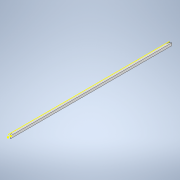
# Autodesk Inventor part: Main
Saved by Autodesk Inventor 2020.1 (Build 241239000, 239)
## iProperties
Created: 2020-02-04
Part Number: Main
Material: Generic
Document SubType Name: Modeling
Designer: super
Density: 1 g/cm^3
Appearance: Default
Author: super
Autodesk Inventor part; units mm, degrees
ref_plane "YZ Plane" through (0, 0, 0) normal (1, 0, 0) x (0, 1, 0)
ref_plane "XZ Plane" through (0, 0, 0) normal (0, 1, 0) x (-1, 0, 0)
ref_plane "XY Plane" through (0, 0, 0) normal (0, 0, 1) x (1, 0, 0)
sketch "Sketch1" plane through (0, 0, 0) normal (0, 1, 0) x (-1, 0, 0)
  line L0 (0, 0) -> (0, -412)
  line L1 (0, -412) -> (6.35, -412)
  line L2 (6.35, -412) -> (6.35, 0)
  line L3 (6.35, 0) -> (0, 0)
  dimension "d0" = 412
  dimension "d1" = 6.35
  constraints: 8 end point, 3 perpendicular, 1 vertical
  measures "d0" distance of L0.start L0.end
  measures "d1" distance of L0.end L1.end
extrude "Extrusion1" add sketch "Sketch1" along normal blind 6.35
sketch "Sketch2" plane through (0, 6.35, 0) normal (0, 1, 0) x (1, 0, 0)
  point P0 (0, 0)
sketch "Sketch3" plane through (-6.35, 0, -412) normal (-1, 0, 0) x (0, 0, 1)
  line L0 (412, 6.35) -> (0, 6.35) projected
  point P0 (412, 0)
sketch "Sketch4" plane through (-6.35, 0, -412) normal (-1, 0, 0) x (0, 0, 1)
  line L0 (412, 6.35) -> (403.5733, 0)
  line L1 (412, 0) -> (0, 0) projected
  line L2 (412, 6.35) -> (422.5514, 6.35) construction
  line L3 (403.5733, 0) -> (412, 0)
  line L4 (412, 0) -> (412, 6.35)
  dimension "d6" = 143
  constraints: 8 end point, 2 point on line, 1 collinear, 1 equal length, 1 horizontal, 1 perpendicular
  measures "d6" angle of L0 L2
extrude "Extrusion2" cut sketch "Sketch4" against normal blind 10
sketch "Sketch5" plane through (-6.35, 0, -412) normal (-1, 0, 0) x (0, 0, 1)
  line L0 (0, 6.35) -> (8.4267, 0)
  line L1 (0, 6.35) -> (10.5514, 6.35) construction
  line L2 (8.4267, 0) -> (0, 0)
  line L3 (0, 6.35) -> (412, 6.35) projected
  line L4 (0, 0) -> (0, 6.35)
  point P0 (412, 0)
  dimension "d9" = 37
  constraints: 8 end point, 1 equal length, 1 horizontal, 1 parallel, 1 perpendicular
  measures "d9" angle of L0 L1
extrude "Extrusion3" cut sketch "Sketch5" against normal blind 10
sketch "Sketch6" plane through (-6.35, 0, -403.5733) normal (-1, 0, 0) x (0, 0, 1)
  line L0 (403.5733, 6.35) -> (-8.4267, 6.35) projected
  line L1 (403.5733, 6.35) -> (403.5733, 0)
  line L2 (403.5733, 6.35) -> (395.1465, 0) projected
  line L3 (403.5733, 0) -> (395.1465, 0)
  line L4 (395.1465, 0) -> (403.5733, 6.35)
  constraints: 6 end point, 1 collinear, 1 perpendicular, 1 vertical
extrude "Extrusion4" add sketch "Sketch6" against normal blind 6.35
sketch "Sketch7" plane through (-6.35, 6.35, -412) normal (-1, 0, 0) x (0, 0, 1)
  line L0 (8.4267, -6.35) -> (412, -6.35) projected
  line L1 (8.4267, -6.35) -> (0, -6.35)
  line L2 (0, 0) -> (412, 0) projected
  line L3 (0, -6.35) -> (0, 0)
  line L4 (0, 0) -> (8.4267, -6.35)
  constraints: 6 end point, 1 horizontal, 1 perpendicular
extrude "Extrusion5" add sketch "Sketch7" against normal blind 6.35
sketch "Sketch8" plane through (0, 6.35, 0) normal (0, 1, 0) x (1, 0, 0)
  line L0 (-6.35, 0) -> (0, 0) projected
  line L1 (0, 0) -> (-6.35, 8.4267)
  line L2 (0, 0) -> (10.5514, 0) construction
  line L3 (-6.35, 8.4267) -> (-6.35, 0)
  line L4 (-6.35, 0) -> (0, 0)
  dimension "d16" = 127
  constraints: 8 end point, 1 collinear, 1 equal length, 1 horizontal, 1 perpendicular
  measures "d16" angle of L2 L1
extrude "Extrusion6" cut sketch "Sketch8" against normal blind 10
sketch "Sketch9" plane through (0, 6.35, 0) normal (0, 1, 0) x (1, 0, 0)
  line L0 (0, 412) -> (-6.3367, 403.5909)
  line L1 (0, 412) -> (10.5293, 412) construction
  line L2 (-6.3367, 403.5909) -> (-6.3367, 412)
  line L3 (0, 0) -> (0, 412) projected
  line L4 (-6.3367, 412) -> (0, 412)
  dimension "d19" = 127
  constraints: 8 end point, 1 equal length, 1 horizontal, 1 parallel, 1 point on line
  measures "d19" angle of L0 L1
extrude "Extrusion7" cut sketch "Sketch9" against normal blind 10
body "Solid1"
